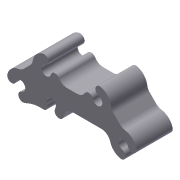
# Autodesk Inventor part: am-0212
Saved by Autodesk Inventor 2013 (Build 170138000, 138)
## iProperties
Category: Chassis
Created: 2010-11-16
Part Number: am-0212
Document SubType Name: Modeling
Designer: Autodesk Inc.
Density: 2.71 g/cm^3
Catalog Web Link: http://www.andymark.com/ProductDetails.asp?ProductCode=am%2D0212
Description: Corner Connect piece for use in C-Base Drive Chassis  Eight of these pieces come standard in the C-Base.
Vendor: AndyMark
Material: Aluminum-6061
Mass: 107.28 g
Surface Area: 111.45 cm^2
Volume: 39.5869 cm^3
Author: Autodesk Inc.
Title: Autodesk Inc.
Autodesk Inventor part; units mm, degrees
ref_plane "YZ Plane" through (0, 0, 0) normal (1, 0, 0) x (0, 1, 0)
ref_plane "XZ Plane" through (0, 0, 0) normal (0, 1, 0) x (-1, 0, 0)
ref_plane "XY Plane" through (0, 0, 0) normal (0, 0, 1) x (1, 0, 0)
sketch "Sketch1" plane through (0, 0, 0) normal (0, 0, 1) x (1, 0, 0)
  arc A0 (63.3108, 19.3076) -> (65.1069, 15.7154) centre (69.597, 20.2056) ccw
  arc A1 (63.3108, 19.3076) -> (56.1947, 27.2004) centre (53.8815, 17.9605) ccw
  arc A2 (56.1947, 27.2004) -> (54.6834, 21.1637) centre (55.439, 24.182) ccw
  arc A3 (50.6775, 17.1623) -> (54.6834, 21.1637) centre (53.8815, 17.9605) ccw
  arc A4 (50.6775, 17.1623) -> (44.9626, 17.9641) centre (47.6583, 16.4101) ccw
  arc A5 (39.4613, 14.7855) -> (44.9626, 17.9641) centre (39.4613, 21.1355) ccw
  line L0 (32.3778, 14.7855) -> (39.4613, 14.7855)
  arc A6 (26.8779, 17.9617) -> (32.3778, 14.7855) centre (32.3778, 21.1355) ccw
  arc A7 (26.8779, 17.9617) -> (21.1641, 17.1604) centre (24.1829, 16.4065) ccw
  arc A8 (17.1604, 21.1641) -> (21.1641, 17.1604) centre (17.9605, 17.9605) ccw
  arc A9 (17.1604, 21.1641) -> (15.6526, 27.2017) centre (16.4065, 24.1829) ccw
  arc A10 (15.6526, 27.2017) -> (8.5312, 19.3076) centre (17.9605, 17.9605) ccw
  arc A11 (6.7352, 15.7154) -> (8.5312, 19.3076) centre (2.2451, 20.2056) ccw
  line L1 (2.2451, 11.2253) -> (6.7352, 15.7154)
  arc A12 (-1.347, 9.4293) -> (2.2451, 11.2253) centre (-2.2451, 15.7154) ccw
  arc A13 (-1.347, 9.4293) -> (-9.2412, 2.3079) centre (0, 0) ccw
  arc A14 (-9.2412, 2.3079) -> (-3.2036, 0.8001) centre (-6.2224, 1.554) ccw
  arc A15 (0.8001, -3.2036) -> (-3.2036, 0.8001) centre (0, 0) ccw
  arc A16 (0.8001, -3.2036) -> (2.3079, -9.2412) centre (1.554, -6.2224) ccw
  arc A17 (2.3079, -9.2412) -> (4.0839, -8.6051) centre (0, 0) ccw
  arc A18 (15.7006, -6.4053) -> (4.0839, -8.6051) centre (14.0949, -29.6986) ccw
  arc A19 (15.7006, -6.4053) -> (18.5812, -1.6996) centre (15.9135, -3.3011) ccw
  arc A20 (24.2432, -1.6996) -> (18.5812, -1.6996) centre (21.4122, 0) ccw
  arc A21 (24.2432, -1.6996) -> (29.5786, -4.9026) centre (26.9109, -3.3011) ccw
  arc A22 (29.5786, -4.9026) -> (30.5871, -2.5587) centre (21.4122, 0) ccw
  arc A23 (36.7037, 2.0855) -> (30.5871, -2.5587) centre (36.7037, -4.2645) ccw
  line L2 (56.5506, 2.0855) -> (36.7037, 2.0855)
  arc A24 (62.6672, -2.5587) -> (56.5506, 2.0855) centre (56.5506, -4.2645) ccw
  arc A25 (62.6672, -2.5587) -> (69.5342, -9.2412) centre (71.842, 0) ccw
  arc A26 (69.5342, -9.2412) -> (71.042, -3.2036) centre (70.2881, -6.2224) ccw
  arc A27 (75.0457, 0.8001) -> (71.042, -3.2036) centre (71.842, 0) ccw
  arc A28 (75.0457, 0.8001) -> (81.0832, 2.3079) centre (78.0644, 1.554) ccw
  arc A29 (81.0832, 2.3079) -> (73.1891, 9.4293) centre (71.842, 0) ccw
  arc A30 (69.597, 11.2253) -> (73.1891, 9.4293) centre (74.0871, 15.7154) ccw
  line L3 (65.1069, 15.7154) -> (69.597, 11.2253)
  constraints: 62 point on circle, 31 centre point, 8 end point, 1 horizontal
extrude "Extrusion1" add sketch "Sketch1" against normal blind 25.273
body "Solid1"
